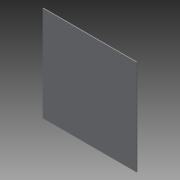
# Autodesk Inventor part: spin4v23.brd_Routing Outlines1
Saved by Autodesk Inventor 2015 SP1 (Build 190203100, 203)
## iProperties
Created: 2015-06-25
Part Number: spin4v23.brd_Routing Outlines1
Material: Generic
Document SubType Name: Modeling
Designer: Patrick
Density: 1 g/cm^3
Appearance: Default
Author: Patrick
Autodesk Inventor part; units mm, degrees
ref_plane "YZ Plane" through (0, 0, 0) normal (1, 0, 0) x (0, 1, 0)
ref_plane "XZ Plane" through (0, 0, 0) normal (0, 1, 0) x (-1, 0, 0)
ref_plane "XY Plane" through (0, 0, 0) normal (0, 0, 1) x (1, 0, 0)
sketch "Routing Outline1_Bottom" plane through (0, 0, 0) normal (0, 0, 1) x (1, 0, 0)
  line L0 (-117, -116.7) -> (113, -116.7)
  line L1 (113, -116.7) -> (113, 116.7)
  line L2 (113, 116.7) -> (-117, 116.7)
  line L3 (-117, 116.7) -> (-117, -116.7)
  line L4 (-117, 0) -> (113, 0) construction
  line L5 (-2, 116.7) -> (-2, -116.7) construction
  line L6 (0, -163.38) -> (0, 163.38) projected
  point P0 (-2, 0)
  point P1 (0, 116.7)
  dimension "d6" = 116.7
  dimension "d10" = 115
  dimension "d11" = 2
  constraints: 12 end point, 5 midpoint, 2 horizontal, 2 point on line, 2 vertical
  measures "d6" distance of L2.end L4.start
  measures "d10" distance of L2.end L5.start
  measures "d11" distance of L5.start point (0, 116.7)
extrude "Extrusion1" add sketch "Routing Outline1_Bottom" along normal blind 2
body "Solid1"
